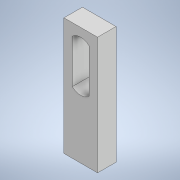
# Autodesk Inventor part: PiezaAux
Saved by Autodesk Inventor 2022 (Build 260153000, 153)
## iProperties
Created: 2022-11-15
Part Number: PiezaAux
Material: Genérico
Document SubType Name: Modeling
Designer: Usuario
Density: 1 g/cm^3
Appearance: Valor por defecto
Author: Usuario
Autodesk Inventor part; units mm, degrees
ref_plane "YZ Plane" through (0, 0, 0) normal (1, 0, 0) x (0, 1, 0)
ref_plane "XZ Plane" through (0, 0, 0) normal (0, 1, 0) x (-1, 0, 0)
ref_plane "XY Plane" through (0, 0, 0) normal (0, 0, 1) x (1, 0, 0)
sketch "Boceto1" plane through (0, 0, 0) normal (0, 0, 1) x (1, 0, 0)
  line L0 (-50, 0) -> (-50, -10)
  line L1 (-50, -10) -> (-45, -10)
  line L2 (-50, -10) -> (50, -10)
  line L3 (-45, -10) -> (-45, 0)
  line L4 (0, 0) -> (-50, 0)
  arc A0 (-45, 0) -> (-45, -10) centre (-45, -5) ccw
  line L5 (-50, -5) -> (-25, -5)
  line L6 (-25, -5) -> (-25, 25)
  line L7 (-25, 25) -> (-15, 25)
  line L8 (-15, 25) -> (-15, -5)
  line L9 (-15, -5) -> (-25, -5)
  line L10 (-20, 25) -> (-20, 5)
  line L11 (-22.5, 7.5) -> (-17.5, 7.5)
  line L12 (-17.5, 7.5) -> (-17.5, 22.5)
  line L13 (-17.5, 22.5) -> (-22.5, 22.5)
  line L14 (-22.5, 22.5) -> (-22.5, 7.5)
  line L15 (-22.5, 7.5) -> (-17.5, 22.5) construction
  line L16 (-17.5, 7.5) -> (-22.5, 22.5) construction
  line L17 (-22.5, 22.5) -> (-22.5, 21.5)
  line L18 (-22.5, 21.5) -> (-17.5, 21.5)
  line L19 (-22.5, 15) -> (-17.5, 15)
  arc A1 (-17.5, 21.5) -> (-22.5, 21.5) centre (-20, 18.875) ccw
  arc A2 (-22.5, 8.5) -> (-17.5, 8.5) centre (-20, 11.125) ccw
  line L20 (-25, -5) -> (-20, -5)
  line L21 (-20, -5) -> (-20, -10)
  line L22 (-20, -10) -> (-25, -10)
  line L23 (-25, -10) -> (-25, -5)
  line L24 (-25, 0) -> (-15, 0)
  line L25 (-15, -5) -> (-15, -10)
  point P0 (0, -10)
  point P1 (-20, 15)
  point P2 (-50, -5)
  point P3 (-20, 22.5)
  point P4 (-20, 7.5)
  point P5 (-22.5, 8.5)
  point P6 (-17.5, 8.5)
  point P7 (-20, -5)
  point P8 (-17.5, 8.5)
  point P9 (-22.5, 8.5)
  dimension "d0" = 5
  dimension "d1" = 25
  dimension "d2" = 30
  dimension "d3" = 10
  dimension "d4" = 20
  dimension "d5" = 5
  dimension "d6" = 15
  dimension "d7" = 1
  constraints: 52 end point, 10 point on line, 9 perpendicular, 7 midpoint, 7 point on circle, 4 parallel, 3 centre point, 3 horizontal, 3 symmetric about line, 2 tangent, 1 vertical, 1 other
  measures "d0" distance of L0.end L1.end
  measures "d1" distance of L5.start L5.end
  measures "d2" distance of L5.end L6.end
  measures "d3" distance of L6.end L7.end
  measures "d4" distance of L10.start L10.end
  measures "d5" distance of L13.end L12.end
  measures "d6" distance of L12.end L11.end
  measures "d7" distance of L13.end L17.end
extrude "Extrusión1" add sketch "Boceto1" against normal blind 5.5 contours L13 L12 A1 | A1 L14 L13 | L6 L7 L8 L4 | L4 L8 L9 L6 | L23 L9 L21 L2 | L21 L9 L25 L2 | A2 L12 L11 | L11 L14 A2
